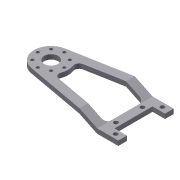
# Autodesk Inventor part: Arm
Saved by Autodesk Inventor 2011 (Build 150239000, 239)
## iProperties
Created: 2010-11-26
Part Number: Arm
Document SubType Name: Modeling
Designer: Milton
Density: 2.71 g/cm^3
Mass: 8.46923 g
Surface Area: 34.1026 cm^2
Volume: 3.12518 cm^3
Material: Aluminum-6061
Author: Milton
Autodesk Inventor part; units mm, degrees
ref_plane "YZ Plane" through (0, 0, 0) normal (1, 0, 0) x (0, 1, 0)
sketch "Sketch1" plane through (0, 0, 0) normal (0, 0, 1) x (1, 0, 0)
  circle A0 centre (66.3461, 11.6829) radius 1.35
  circle A1 centre (66.349, 28.6829) radius 1.35
  circle A2 centre (72.6461, 5.1829) radius 1.35
  circle A3 centre (72.649, 35.1829) radius 1.35
  line L0 (77.149, 32.3829) -> (77.149, 37.9829)
  line L1 (77.149, 7.9829) -> (77.149, 2.3829)
  line L2 (77.149, 32.3829) -> (69.149, 32.3829)
  line L3 (69.149, 32.3829) -> (69.149, 7.9829)
  line L4 (69.149, 7.9829) -> (77.149, 7.9829)
  circle A4 centre (16.149, 20.1829) radius 4.5
  line L5 (77.149, 37.9829) -> (52.149, 37.9829)
  arc A5 (14.1608, 31.0018) -> (14.1608, 9.3641) centre (16.149, 20.1829) ccw
  line L6 (52.149, 37.9829) -> (14.1608, 31.0018)
  line L7 (77.149, 2.3829) -> (52.149, 2.3829)
  line L8 (52.149, 2.3829) -> (14.1608, 9.3641)
  line L9 (63.549, 7.9829) -> (63.549, 32.3829)
  line L10 (63.549, 32.3829) -> (52.149, 32.3829)
  line L11 (52.149, 32.3829) -> (24.5301, 27.3073)
  line L12 (52.149, 7.9829) -> (63.549, 7.9829)
  line L13 (52.149, 7.9829) -> (24.5301, 13.0585)
  arc A6 (24.5301, 13.0585) -> (24.5301, 27.3073) centre (16.149, 20.1829) ccw
  point P0 (0, 0)
  dimension "d2" = 9
  dimension "d26" = 8
  dimension "d27" = 8
  dimension "d29" = 2.8
  dimension "d30" = 6.3
  dimension "d31" = 6.3
  dimension "d32" = 25
  dimension "d33" = 22
  dimension "d34" = 25
  dimension "d43" = 5.6
  dimension "d44" = 5.6
  dimension "d46" = 5.6
  dimension "d47" = 11.4
  dimension "d48" = 11.4
  constraints: 28 end point, 7 centre point, 5 parallel, 4 point on circle, 2 coincident, 2 perpendicular, 2 tangent
  measures "d2" diameter of A4
  measures "d26" distance of L0.start L2.end
  measures "d27" distance of L3.end L1.start
  measures "d29" distance from line of L3 A1.centre
  measures "d30" horizontal distance of A1.centre A3.centre
  measures "d31" horizontal distance of A2.centre A0.centre
  measures "d32" distance of L0.end L5.end
  measures "d33" diameter of A5
  measures "d34" distance of L1.end L7.end
  measures "d43" distance between parallel lines of L5 L10
  measures "d44" distance between parallel lines of L3 L9
  measures "d46" distance between parallel lines of L7 L12
  measures "d47" distance of L9.end L10.end
  measures "d48" distance of L12.start L9.start
extrude "Extrusion1" add sketch "Sketch1" along normal blind 3
ref_plane "Work Plane1" through (47.9215, -19.8251, -5.5) normal (0, 0, 1) x (1, 0, 0)
sketch "Sketch5" plane through (0, 0, 0) normal (0, 0, -1) x (-1, 0, 0)
  line L0 (-52.149, 7.9829) -> (-63.549, 7.9829) projected
  line L1 (-63.549, 32.3829) -> (-52.149, 32.3829) projected
  circle A0 centre (-72.6461, 5.1829) radius 1.35 projected
  circle A1 centre (-66.349, 28.6829) radius 1.35 projected
  circle A2 centre (-66.3461, 11.6829) radius 1.35 projected
  circle A3 centre (-72.649, 35.1829) radius 1.35 projected
  line L2 (-77.149, 32.3829) -> (-77.149, 37.9829) projected
  line L3 (-77.149, 2.3829) -> (-77.149, 7.9829) projected
  line L4 (-77.149, 37.9829) -> (-52.149, 37.9829) projected
  line L5 (-77.149, 32.3829) -> (-69.149, 32.3829)
  line L6 (-69.149, 32.3829) -> (-69.149, 7.9829)
  line L7 (-69.149, 7.9829) -> (-77.149, 7.9829)
  line L8 (-77.149, 7.9829) -> (-77.149, 2.3829)
  line L9 (-77.149, 2.3829) -> (-52.149, 2.3829)
  line L10 (-52.149, 2.3829) -> (-52.149, 7.9829)
  line L11 (-63.549, 7.9829) -> (-63.549, 32.3829)
  line L12 (-52.149, 32.3829) -> (-52.149, 37.9829)
  line L13 (-63.549, 32.3829) -> (-52.149, 32.3829)
  line L14 (-52.149, 37.9829) -> (-77.149, 37.9829)
  line L15 (-77.149, 32.3829) -> (-77.149, 37.9829)
  circle A4 centre (-72.649, 35.1829) radius 1.35
  circle A5 centre (-66.349, 28.6829) radius 1.35
  circle A6 centre (-66.3461, 11.6829) radius 1.35
  circle A7 centre (-72.6461, 5.1829) radius 1.35
  point P0 (0, 0)
  dimension "d49" = 2.7
  dimension "d50" = 2.7
  constraints: 22 end point, 5 perpendicular, 4 centre point, 4 coincident, 4 parallel, 2 collinear, 2 concentric
  measures "d49" diameter of A6
  measures "d50" diameter of A7
ref_plane "Work Plane2" through (55.1914, -9.495, -5.5) normal (0, 0, 1) x (1, 0, 0)
extrude "Extrusion5" add sketch "Sketch5" along normal up to surface (5.5 mm away)
sketch "Sketch6" plane through (52.149, 2.3829, 3) normal (0, -1, 0) x (1, 0, 0)
  line L0 (0, -3) -> (0, -8.5) projected
  line L1 (25, -8.5) -> (0, -8.5) projected
  line L2 (25, -8.5) -> (25, 0) projected
  line L3 (0, -3) -> (11.4, -8.5)
  line L4 (11.4, -8.5) -> (0, -8.5)
  line L5 (0, -8.5) -> (0, -3)
  line L6 (0, 0) -> (11.4, -5.5)
  line L7 (11.4, -8.5) -> (11.4, 0) projected
  line L8 (11.4, -5.5) -> (25, -5.5)
  line L9 (25, -8.5) -> (25, 0) projected
  line L10 (25, -5.5) -> (25, 0)
  line L11 (25, 0) -> (17, 0) projected
  line L12 (25, 0) -> (0, 0)
  point P0 (-52.149, -3)
  constraints: 14 end point, 3 perpendicular, 2 collinear, 2 point on line, 1 parallel
extrude "Extrusion6" cut sketch "Sketch6" against normal through all contours L3 L1 L0 | L6 L12 L7 | L7 L12 L11 L2 L8
fillet "Fillet2" radius 3 4 edges at (63.549, 32.3829, -4) (24.5301, 27.3073, 1.5) (24.5301, 13.0585, 1.5) (63.549, 7.9829, -4)
sketch "Sketch7" plane through (0, 0, 3) normal (0, 0, 1) x (1, 0, 0)
  arc A0 (26.4411, 16.3006) -> (26.4411, 24.0653) centre (16.149, 20.1829) ccw projected
  circle A1 centre (16.149, 28.6829) radius 1
  point P0 (0, 0)
  dimension "d56" = 2
  dimension "d57" = 8.5
  constraints: 1 centre point
  measures "d56" diameter of A1
  measures "d57" distance of A0.centre A1.centre
extrude "Extrusion7" cut sketch "Sketch7" against normal through all
pattern_circular "Circular Pattern1" count 8 over 360 about axis through (16.149, 20.1829, 0) along (0, 0, 1) of "Extrusion7"
body "Solid1"
